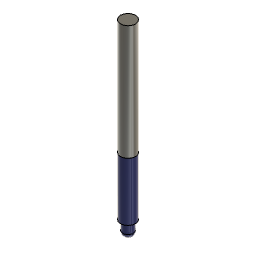
BlueSharpie (Autodesk Fusion 360 design; units mm, degrees)
Autodesk Fusion 360 part; units mm, degrees
sketch "Sketch1" plane through (0, 0, 0) normal (0, 0, 1) x (1, 0, 0)
  circle A0 centre (0, 0) radius 5.55
  dimension "d1" = 11.1
  constraint coincident A0.centre origin
  measures "d1" diameter of A0
extrude "Extrude1" add sketch "Sketch1" along normal blind 85 makes body 1
sphere "SpherePrimitive6" add diameter 11 placed x (1, 0, 0) y (0, 1, 0) z (0, 0, 1) at (16, 156, 0) separate body makes body 2
move_body "Move1" bodies 2 to x (1, 0, 0) y (0, 1, 0) z (0, 0, 1) at (-16, -156, 85)
move_body "MoveFace1" bodies 2 to x (1, 0, 0) y (0, 1, 0) z (0, 0, 1) at (0, 0, -1) on bodies 2
move_body "MoveFace2" bodies 2 to x (1, 0, 0) y (0, 1, 0) z (0, 0, 1) at (0, 0, 1) on bodies 2
combine "Combine1" operation add target body 2 tool bodies 1
cylinder "CylinderPrimitive1" add diameter 11 height 50 placed x (0, 1, 0) y (1, 0, 0) z (0, 0, -1) at (0, 0, 0) bodies 2
delete_face "DeleteFace4" 1 faces at (-0.5476, 5.4727, -33.3333) on bodies 2
cylinder "CylinderPrimitive2" add diameter 11 height 43 placed x (0, 1, 0) y (1, 0, 0) z (0, 0, -1) at (0, 0, 0) bodies 2
cylinder "CylinderPrimitive3" add diameter 7.8 height 7 placed x (0, 1, 0) y (1, 0, 0) z (0, 0, -1) at (0, 0, -43) bodies 2
sphere "SpherePrimitive8" add diameter 7.8 placed x (1, 0, 0) y (0, 1, 0) z (0, 0, 1) at (14, 37, 0) separate body makes body 3
move_body "MoveFace3" bodies 3 to x (1, 0, 0) y (0, 1, 0) z (0, 0, 1) at (-14, -37, -50) on bodies 3
delete_face "DeleteFace5" 1 faces at (-2.7265, -4.7224, 85.7179) on bodies 2
sketch "Sketch13" plane through (0, 0, 0) normal (0, 1, 0) x (1, 0, 0)
